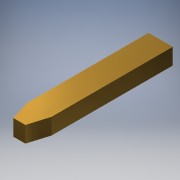
# Autodesk Inventor part: Pin
Saved by Autodesk Inventor 2018.3 (Build 223284000, 284)
## iProperties
Created: 2020-11-16
Part Number: Pin
Material: Generic
Document SubType Name: Modeling
Designer: daanv
Density: 1 g/cm^3
Appearance: Brass - Satin(1)
Author: daanv
Autodesk Inventor part; units mm, degrees
ref_plane "YZ Plane" through (0, 0, 0) normal (1, 0, 0) x (0, 1, 0)
ref_plane "XZ Plane" through (0, 0, 0) normal (0, 1, 0) x (-1, 0, 0)
ref_plane "XY Plane" through (0, 0, 0) normal (0, 0, 1) x (1, 0, 0)
sketch "Sketch1" plane through (0, 0, 0) normal (0, 0, 1) x (1, 0, 0)
  line L0 (0, 3.5) -> (0, 0.5)
  line L1 (0, 0.5) -> (0.15, 0)
  line L2 (0.15, 0) -> (0.45, 0)
  line L3 (0.45, 0) -> (0.6, 0.5)
  line L4 (0.6, 0.5) -> (0.6, 3.5)
  line L5 (0.6, 3.5) -> (0, 3.5)
  point P0 (0, 0)
  dimension "d0" = 3
  dimension "d1" = 0.6
  dimension "d2" = 0.3
  dimension "d3" = 0.5
  dimension "d4" = 0.15
  dimension "d5" = 0.15
  constraints: 12 end point, 2 perpendicular, 1 parallel, 1 vertical
  measures "d0" distance of L0.start L0.end
  measures "d1" distance of L4.end L0.start
  measures "d2" distance of L1.end L2.end
  measures "d3" vertical distance of L1.end L0.end
  measures "d4" horizontal distance of L1.end L0.end
  measures "d5" horizontal distance of L2.end L3.end
extrude "Extrusion1" add sketch "Sketch1" along normal blind 0.4
body "Solid1"
